sample v1 (Autodesk Fusion 360 design; units mm, degrees)
Autodesk Fusion 360 part; units mm, degrees
box "BoxPrimitive1" add length 34.5322 width 45.1485 height 10 placed x (0, 1, 0) y (-1, 0, 0) z (0, 0, 1) at (46.7416, -12.77, 0)
